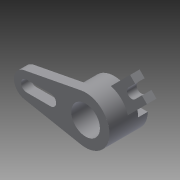
# Autodesk Inventor part: 零件7-21-2
Saved by Autodesk Inventor 2014 (Build 180170000, 170)
## iProperties
Created: 2018-12-21
Part Number: 零件7-21-2
Material: 常规
Document SubType Name: Modeling
Designer: Administrator
Density: 1 g/cm^3
Appearance: 默认
Author: Administrator
Autodesk Inventor part; units mm, degrees
ref_plane "YZ Plane" through (0, 0, 0) normal (1, 0, 0) x (0, 1, 0)
ref_plane "XZ Plane" through (0, 0, 0) normal (0, 1, 0) x (-1, 0, 0)
ref_plane "XY Plane" through (0, 0, 0) normal (0, 0, 1) x (1, 0, 0)
sketch "草图1" plane through (0, 0, 0) normal (0, 1, 0) x (-1, 0, 0)
  circle A0 centre (0, 0) radius 15
  arc A1 (38.5135, -7.8555) -> (38.5135, 7.8555) centre (37, 0) ccw
  line L0 (38.5135, -7.8555) -> (2.8378, -14.7291)
  line L1 (2.8378, 14.7291) -> (39.6131, 7.6437)
  line L2 (50.7291, 0) -> (-22.1307, 0)
  arc A2 (37, -3.5) -> (37, 3.5) centre (37, 0) ccw
  arc A3 (22, 3.5) -> (22, -3.5) centre (22, 0) ccw
  line L3 (37, -3.5) -> (22, -3.5)
  line L4 (22, 3.5) -> (37, 3.5)
  dimension "d0" = 30
  dimension "d1" = 16
  dimension "d2" = 37
  dimension "d3" = 7
  dimension "d4" = 7
  dimension "d5" = 15
  constraints: 10 end point, 8 point on circle, 6 tangent, 4 centre point, 4 point on line, 2 coincident, 1 horizontal, 1 parallel
  measures "d0" diameter of A0
  measures "d1" diameter of A1
  measures "d2" distance of A0.centre A1.centre
  measures "d3" diameter of A2
  measures "d4" diameter of A3
  measures "d5" distance of A2.centre A3.centre
extrude "拉伸1" add sketch "草图1" along normal blind 6 contours L2 A0 | L2 A3 L3 A2 A1 L0 A0 | A0 L1 A1 L2 A2 L4 A3 | A0 L2
sketch "草图2" plane through (0, 6, 0) normal (0, 1, 0) x (1, 0, 0)
  line L0 (-37, 3.5) -> (-22, 3.5) projected
  arc A0 (-22, -3.5) -> (-22, 3.5) centre (-22, 0) ccw projected
  line L1 (-22, -3.5) -> (-37, -3.5) projected
  arc A1 (-37, 3.5) -> (-37, -3.5) centre (-37, 0) ccw projected
  arc A2 (-38.5135, 7.8555) -> (-38.5135, -7.8555) centre (-37, 0) ccw projected
  line L2 (-38.5135, -7.8555) -> (-2.8378, -14.7291) projected
  arc A3 (-2.8378, -14.7291) -> (-2.8378, 14.7291) centre (0, 0) ccw projected
  line L3 (-2.8378, 14.7291) -> (-38.5135, 7.8555) projected
  circle A4 centre (0, 0) radius 15
  constraints: 1 centre point, 1 coincident
extrude "拉伸2" add sketch "草图2" along normal blind 12 contours A3 A4
sketch "草图3" plane through (0, 18, 0) normal (0, 1, 0) x (1, 0, 0)
  circle A0 centre (0, 0) radius 15 projected
  circle A1 centre (0, 0) radius 9
  dimension "d10" = 18
  constraints: 1 centre point, 1 coincident
  measures "d10" diameter of A1
extrude "拉伸3" cut sketch "草图3" against normal blind 20 contours A1
sketch "草图4" plane through (0, 18, 0) normal (0, 1, 0) x (1, 0, 0)
  circle A0 centre (0, 0) radius 9 projected
  circle A1 centre (0, 0) radius 15 projected
  line L0 (9, 0) -> (15, 0)
  line L1 (6.364, 6.364) -> (10.6066, 10.6066)
  dimension "d13" = 45
  constraints: 4 end point, 4 point on circle, 1 horizontal
  measures "d13" angle of L0 L1
extrude "拉伸4" add sketch "草图4" along normal blind 6 contours A0 L1 A1 L0 picked at (12.295, 4.0369)
sketch "草图5" plane through (0, 18, 0) normal (0, 1, 0) x (1, 0, 0)
  arc A0 (10.6066, 10.6066) -> (15, 0) centre (0, 0) ccw projected
  line L0 (15, 0) -> (9, 0) projected
  arc A1 (6.364, 6.364) -> (9, 0) centre (0, 0) ccw projected
  line L1 (0, 0) -> (21.2132, -21.2132) construction
  line L2 (26.5165, -15.9099) -> (14.4889, -3.8823)
  line L3 (3.8823, -14.4889) -> (15.9099, -26.5165)
  line L4 (26.5165, -15.9099) -> (1.7678, -12.3744) construction
  line L5 (12.3744, -1.7678) -> (15.9099, -26.5165) construction
  arc A2 (19.0919, -14.8492) -> (14.8492, -19.0919) centre (16.9706, -16.9706) ccw
  line L6 (14.8492, -19.0919) -> (19.0919, -23.3345)
  line L7 (19.0919, -14.8492) -> (23.3345, -19.0919)
  line L8 (15.9099, -26.5165) -> (19.0919, -23.3345)
  line L9 (23.3345, -19.0919) -> (26.5165, -15.9099)
  point P0 (14.1421, -14.1421)
  dimension "d16" = 45
  dimension "d17" = 15
  dimension "d20" = 6
  constraints: 18 end point, 4 perpendicular, 4 point on circle, 4 point on line, 2 midpoint, 2 tangent, 1 centre point, 1 parallel
  measures "d16" angle of L1 L0
  measures "d17" distance of L4.end L5.start
  measures "d20" diameter of A2
extrude "拉伸5" add sketch "草图5" against normal blind 6
